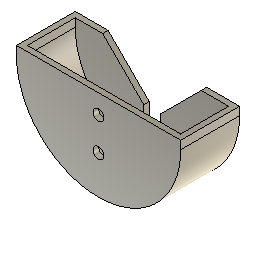
Panel Antenna Mount (Autodesk Fusion 360 design; units mm, degrees)
Autodesk Fusion 360 part; units mm, degrees
sketch "Sketch1" plane through (0, 0, 0) normal (0, 1, 0) x (1, 0, 0)
  arc A0 (28, 0) -> (-28, 0) centre (0, 0) ccw
  line L0 (-28, 0) -> (-28, -3)
  line L1 (0, -1.75) -> (0, -22.5)
  line L2 (28, 0) -> (28, -3)
  line L3 (-30, 0) -> (-30, -3)
  arc A1 (30, 0) -> (-30, 0) centre (0, 0) ccw
  line L4 (30, 0) -> (30, -3)
  line L5 (-30, -3) -> (-28, -3)
  line L6 (28, -3) -> (30, -3)
  line L7 (-3, 29.8496) -> (-3, 12)
  line L8 (-3, 12) -> (-18, -3)
  line L9 (-18, -3) -> (-28, -3)
  line L10 (18, -3) -> (28, -3)
  line L11 (3, 12) -> (18, -3)
  line L12 (3, 29.8496) -> (3, 12)
  line L13 (-18, -3) -> (18, -3)
  circle A2 centre (0, 4) radius 2
  circle A3 centre (0, 16) radius 2
  dimension "d1" = 28
  dimension "d2" = 3
  dimension "d3" = -2
  dimension "d4" = 135
  dimension "d5" = 6
  dimension "d6" = 15
  dimension "d7" = 7
  dimension "d8" = 12
  dimension "d9" = 4
  constraint coincident A0.centre A1.centre
  constraint tangent A0 L0
  constraint vertical L0
  constraint symmetric A0.end L1 A0.start
  constraint symmetric L0.end L1 L2.end
  constraint perpendicular L0 L5
  constraint perpendicular L4 L6
  constraint coincident A1 L7.start
  constraint vertical L7
  constraint perpendicular L0 L9
  constraint symmetric L1 L7.start L12.start
  constraint symmetric L1 L7.end L11.start
  constraint symmetric L1 L8.end L10.start
  constraint equal A2 A3
  constraint vertical A2.centre A3.centre
  constraint vertical A0.centre A2.centre
  measures "d1" radius of A0
  measures "d2" distance of A0.end L0.end
  measures "d4" angle of L7 L8
  measures "d5" distance of L7 L12
  measures "d6" distance of L7.end L9
  measures "d7" distance of L13 A2.centre
  measures "d8" distance of A2.centre A3.centre
  measures "d9" diameter of A2
extrude "Extrude1" add sketch "Sketch1" against normal blind 2
extrude "Extrude2" add sketch "Sketch1" along normal blind 17.5 contours A0 L2 A1 L4 L6 L12 | A0 L0 L3 A1 L5 L7
extrude "Extrude3" add sketch "Sketch1" along normal blind 2 from surface at 17.5 contours A0 L2 L10 L11 L12 | A0 L2 A1 L4 L6 L12 | A0 L0 L7 L8 L9 | A0 L0 L3 A1 L5 L7
fillet "Fillet1" radius 3 2 edges at (3, 0, -28.8442) (-3, 0, -28.8442)
equation "d1 = ( 56 / 2 ) * 1 mm"
